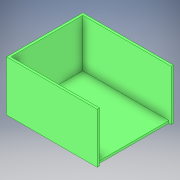
# Autodesk Inventor part: Base_caja
Saved by Autodesk Inventor 2019 (Build 230136000, 136)
## iProperties
Created: 2020-02-05
Part Number: Base_caja
Material: Generic
Document SubType Name: Modeling
Designer: Omar
Density: 1 g/cm^3
Appearance: Default
Author: Omar
Autodesk Inventor part; units mm, degrees
ref_plane "YZ Plane" through (0, 0, 0) normal (1, 0, 0) x (0, 1, 0)
ref_plane "XZ Plane" through (0, 0, 0) normal (0, 1, 0) x (-1, 0, 0)
ref_plane "XY Plane" through (0, 0, 0) normal (0, 0, 1) x (1, 0, 0)
sketch "Sketch1" plane through (0, 0, 0) normal (0, 1, 0) x (-1, 0, 0)
  line L0 (0, 0) -> (120, 0)
  line L1 (120, 0) -> (120, -100)
  line L2 (120, -100) -> (0, -100)
  line L3 (0, -100) -> (0, 0)
  dimension "d0" = 120
  dimension "d1" = 100
  constraints: 8 end point, 2 parallel, 1 horizontal, 1 perpendicular
  measures "d0" distance of L1.end L2.end
  measures "d1" distance of L0.end L1.end
extrude "Extrusion1" add sketch "Sketch1" along normal blind 3.18
sketch "Sketch2" plane through (0, 0, 0) normal (0, 1, 0) x (-1, 0, 0)
  line L0 (120, 0) -> (0, 0) projected
  line L1 (0, 0) -> (0, -100) projected
  line L2 (0, -100) -> (120, -100) projected
  line L3 (120, -100) -> (120, 0) projected
  line L4 (-3.18, 0) -> (123.18, 0)
  line L5 (123.18, 0) -> (123.18, 3.18)
  line L6 (123.18, 3.18) -> (-3.18, 3.18)
  line L7 (-3.18, 3.18) -> (-3.18, 0)
  line L8 (123.18, -100) -> (-3.18, -100)
  line L9 (-3.18, -100) -> (-3.18, -103.18)
  line L10 (-3.18, -103.18) -> (123.18, -103.18)
  line L11 (123.18, -103.18) -> (123.18, -100)
  line L12 (123.18, 0) -> (120, 0)
  line L13 (120, 0) -> (120, -100)
  line L14 (120, -100) -> (123.18, -100)
  line L15 (123.18, -100) -> (123.18, 0)
  dimension "d4" = 3.18
  dimension "d5" = 3.18
  dimension "d6" = 3.18
  dimension "d7" = 3.18
  constraints: 24 end point, 6 parallel, 4 collinear, 3 horizontal, 3 perpendicular, 2 point on line
  measures "d4" distance between parallel lines of L3 L5
  measures "d5" distance between parallel lines of L1 L7
  measures "d6" distance between parallel lines of L4 L6
  measures "d7" distance of L0.start L12.start
extrude "Extrusion2" add sketch "Sketch2" along normal blind 70 contours L4 L15 L8 L3 | L0 L4 L7 L6 L5 | L8 L11 L10 L9 L2
body "Solid1"
